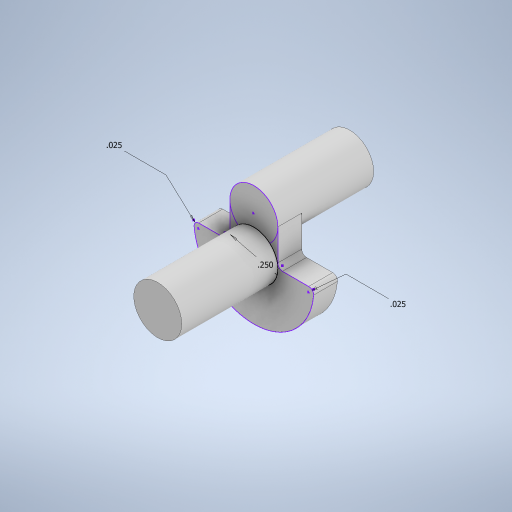
# Autodesk Inventor part: Crankshaft
Saved by Autodesk Inventor 2023 (Build 270158000, 158)
## iProperties
Created: 2022-11-21
Part Number: Crankshaft
Material: Generic
Document SubType Name: Modeling
Designer: tommy
Density: 1 g/cm^3
Appearance: Default
Author: tommy
Autodesk Inventor part; units mm, degrees
ref_plane "YZ Plane" through (0, 0, 0) normal (1, 0, 0) x (0, 1, 0)
ref_plane "XZ Plane" through (0, 0, 0) normal (0, 1, 0) x (-1, 0, 0)
ref_plane "XY Plane" through (0, 0, 0) normal (0, 0, 1) x (1, 0, 0)
sketch "Sketch1" plane through (0, 0, 0) normal (0, 0, 1) x (1, 0, 0)
  circle A0 centre (0, 4.7625) radius 3.175
  arc A1 (-7.9074, -0.6902) -> (7.9074, -0.6902) centre (0, 0) ccw
  line L0 (3.175, 4.7625) -> (3.175, 0.635)
  line L1 (3.81, 0) -> (7.2748, 0)
  line L2 (-3.175, 4.7625) -> (-3.175, 0.635)
  line L3 (-3.81, 0) -> (-7.2748, 0)
  arc A2 (-7.2748, 0) -> (-7.9074, -0.6902) centre (-7.2748, -0.635) ccw
  arc A3 (-3.81, 0) -> (-3.175, 0.635) centre (-3.81, 0.635) ccw
  arc A4 (3.175, 0.635) -> (3.81, 0) centre (3.81, 0.635) ccw
  arc A5 (7.9074, -0.6902) -> (7.2748, 0) centre (7.2748, -0.635) ccw
  circle A6 centre (0, 0) radius 3.175
  circle A7 centre (0, 4.7625) radius 3.175
  point P0 (-3.175, 0)
  point P1 (-7.9375, 0)
  point P2 (7.9375, 0)
  dimension "d2" = 0.635
  dimension "d3" = 0.635
  dimension "d4" = 6.35
  constraints: 14 point on circle, 9 tangent, 8 end point, 7 centre point, 6 point on line, 3 coincident, 2 equal radius, 2 perpendicular, 1 horizontal alignment, 1 vertical, 2 other
  measures "d2" radius of A2
  measures "d3" radius of A5
  measures "d4" diameter of A6
extrude "Extrusion1" add sketch "Sketch1" along normal blind 12.7 contours A6 A0 | A0 A6 picked at (-0.105, -1.5684) picked at (-0.2525, 2.1472)
extrude "Extrusion2" add sketch "Sketch1" against normal blind 3.175
extrude "Extrusion3" add sketch "Sketch1" against normal blind 12.7 contours A0 A6 | A0 A6 picked at (0, 6.3346) picked at (-0.2525, 2.1472)
body "Solid1"
